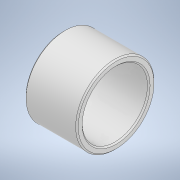
# Autodesk Inventor part: WSSS-12-10-8
Saved by Autodesk Inventor 2020 (Build 240168000, 168)
## iProperties
Created: 2021-09-10
Part Number: WSSS-12-10-8
Material: ステンレス鋼 AISI 304
Document SubType Name: Modeling
Designer: naoki
Density: 6.94202 g/cm^3
Appearance: サテン
Description: 既製品
Mass: 1.9 g
Surface Area: 6.05841 cm^2
Volume: 0.273696 cm^3
Author: Naoki Iwasawa
Comments: https://jp.misumi-ec.com/vona2/detail/110302677010/?HissuCode=WSSS12-10-8
Autodesk Inventor part; units mm, degrees
ref_plane "YZ Plane" through (0, 0, 0) normal (1, 0, 0) x (0, 1, 0)
ref_plane "XZ Plane" through (0, 0, 0) normal (0, 1, 0) x (-1, 0, 0)
ref_plane "XY Plane" through (0, 0, 0) normal (0, 0, 1) x (1, 0, 0)
sketch "スケッチ1" plane through (0, 0, 0) normal (0, 1, 0) x (-1, 0, 0)
  line L0 (0, 3.2045) -> (0, -8.6364) construction
  line L1 (6.7273, 0) -> (-4.6136, 0) construction
  line L2 (-4, -6) -> (-3.8, -6) construction
  line L3 (4, -6) -> (4, -5.8) construction
  line L4 (4, -5) -> (3.8, -5) construction
  line L5 (-4, -5) -> (-4, -5.2) construction
  line L6 (-4, -6) -> (4, -5) construction
  line L7 (4, -6) -> (-4, -5) construction
  line L8 (4, -5.8) -> (3.8, -6)
  line L9 (4, -5.5) -> (-4, -5.5) construction
  line L10 (4, -5.2) -> (3.8, -5)
  line L11 (-4, -5.8) -> (-3.8, -6)
  line L12 (-4, -5.2) -> (-3.8, -5)
  line L13 (4, -5.2) -> (4, -5) construction
  line L14 (3.8, -5) -> (-3.8, -5)
  line L15 (4, -5.8) -> (4, -5.2)
  line L16 (3.8, -6) -> (4, -6) construction
  line L17 (-4, -5.8) -> (-4, -6) construction
  line L18 (-3.8, -6) -> (0, -6)
  line L19 (-4, -5.2) -> (-4, -5.8)
  line L20 (-3.8, -5) -> (-4, -5) construction
  line L21 (0, -6) -> (3.8, -6)
  point P0 (0, 0)
  point P1 (0, -5.5)
  dimension "d1" = 8
  dimension "d2" = 5
  dimension "d3" = 0.2
  dimension "d4" = 0.2
  dimension "d5" = 1
  constraints: 44 end point, 21 parallel, 12 perpendicular, 6 symmetric about line, 5 horizontal, 4 point on line, 2 midpoint, 1 vertical
  measures "d1" distance of L2.start L3.start
  measures "d2" distance between parallel lines of L1 L4
  measures "d3" distance from line of L3 L8.end
  measures "d4" distance of L3.end L3.start
  measures "d5" distance between parallel lines of L14 L21
revolve "回転1" add sketch "スケッチ1" angle 360 about axis through (-6.7273, 0, 0) along (1, 0, 0)
equation "\"d4\" = d3"
